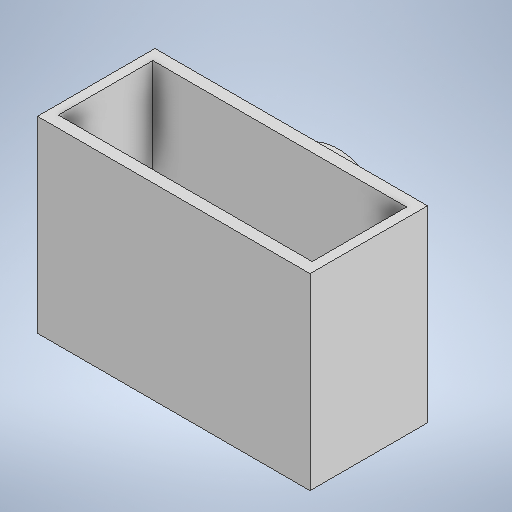
# Autodesk Inventor part: Attache servomoteur_bogie
Saved by Autodesk Inventor 2026.2 (Build 302298010, 298A)
## iProperties
Created: 2026-03-22
Part Number: Attache servomoteur_bogie
Material: Générique
Document SubType Name: Modeling
Designer: Genon
Density: 1 g/cm^3
Appearance: Par défaut
Author: Genon
Autodesk Inventor part; units mm, degrees
ref_plane "YZ Plane" through (0, 0, 0) normal (1, 0, 0) x (0, 1, 0)
ref_plane "XZ Plane" through (0, 0, 0) normal (0, 1, 0) x (-1, 0, 0)
ref_plane "XY Plane" through (0, 0, 0) normal (0, 0, 1) x (1, 0, 0)
sketch "Esquisse1" plane through (0, 0, 0) normal (0, 1, 0) x (-1, 0, 0)
  line L0 (0, 0) -> (0, 2.45)
  line L1 (0, 0) -> (2.45, 0) construction
  line L2 (0, 2.45) -> (27, 2.45)
  line L3 (27, 2.45) -> (27, 22.55)
  line L4 (27, 22.55) -> (-27, 22.55)
  line L5 (-27, 22.55) -> (-27, 2.45)
  line L6 (-27, 2.45) -> (0, 2.45)
  line L7 (0, 0) -> (29, 0)
  line L8 (29, 0) -> (29, 25)
  line L9 (29, 25) -> (-29, 25)
  line L10 (-29, 25) -> (-29, 0)
  line L11 (-29, 0) -> (0, 0)
  dimension "d0" = 2.45
  dimension "d1" = 90
  dimension "d2" = 27
  dimension "d3" = 20.1
  dimension "d4" = 54
  dimension "d5" = 29
  dimension "d6" = 25
  dimension "d7" = 58
  constraints: 24 end point, 6 perpendicular, 4 horizontal, 2 parallel, 1 point on line, 1 vertical
  measures "d0" distance of L0.start L0.end
  measures "d1" angle of L1 L0
  measures "d2" distance of L0.end L2.end
  measures "d3" distance of L2.end L3.end
  measures "d4" distance of L3.end L4.end
  measures "d5" distance of L0.start L7.end
  measures "d6" distance of L7.end L8.end
  measures "d7" distance of L8.end L9.end
extrude "Extrusion1" add sketch "Esquisse1" along normal blind 40
sketch "Esquisse2" plane through (29, 0, 0) normal (0, 0, -1) x (-1, 0, 0)
  line L0 (29, 0) -> (29, 40)
  line L1 (58, 40) -> (0, 40) projected
  line L2 (0, 0) -> (0, 40) projected
  line L3 (0, 20) -> (58, 20)
  line L4 (58, 0) -> (58, 40) projected
  circle A0 centre (29, 20) radius 10
  circle A1 centre (29, 20) radius 11
  dimension "d10" = 20
  dimension "d11" = 22
  constraints: 4 end point, 4 midpoint, 2 centre point, 1 coincident
  measures "d10" diameter of A0
  measures "d11" diameter of A1
extrude "Extrusion2" add sketch "Esquisse2" along normal blind 10 contours A1 L3 A0 L0 | L0 A0 L3 A1 | A1 L0 A0 L3 | L3 A0 L0 A1
sketch "Esquisse3" plane through (0, 0, 0) normal (0, 1, 0) x (-1, 0, 0)
  line L0 (-11, -10) -> (11, -10) projected
  line L1 (0, -10) -> (0, -5)
  point P0 (0, 0)
  dimension "d14" = 5
  constraints: 2 end point, 1 coincident, 1 midpoint, 1 vertical
  measures "d14" distance of L1.start L1.end
hole "Perçage1" at (0, 0, -5) direction (0, 1, 0) diameter 4 end through all
sketch "Esquisse4" plane through (0, 0, 0) normal (0, -1, 0) x (1, 0, 0)
  line L0 (27, 2.45) -> (27, 22.55) projected
  line L1 (27, 22.55) -> (-27, 22.55) projected
  line L2 (-27, 2.45) -> (27, 2.45) projected
  line L3 (-27, 22.55) -> (-27, 2.45) projected
  line L4 (27, 22.55) -> (21, 22.55)
  line L5 (27, 22.55) -> (33, 22.55) construction
  line L6 (21, 22.55) -> (21, 2.45)
  line L7 (-27, 22.55) -> (-21, 22.55)
  line L8 (-21, 22.55) -> (-21, 2.45)
  point P0 (0, 0)
  dimension "d22" = 6
  dimension "d23" = 180
  dimension "d24" = 6
  constraints: 10 end point, 3 point on line, 2 horizontal, 2 perpendicular, 1 collinear
  measures "d22" distance of L0.end L4.end
  measures "d23" angle of L4 L5
  measures "d24" distance of L1.end L7.end
extrude "Extrusion3" add sketch "Esquisse4" against normal blind 16.4 contours L2 L6 L1 L0 | L2 L3 L1 L8
sketch "Esquisse5" plane through (0, 16.4, 0) normal (0, 1, 0) x (1, 0, 0)
  line L0 (-21, -22.55) -> (-21, -2.45) projected
  line L1 (-21, -22.55) -> (-21, -12.5)
  line L2 (-21, -12.5) -> (-21, -11.5)
  line L3 (-27, -22.55) -> (-27, -2.45) projected
  line L4 (-21, -11.5) -> (-27, -11.5)
  line L5 (-21, -12.5) -> (-21, -13.5)
  line L6 (-21, -13.5) -> (-27, -13.5)
  line L7 (0, -14.9752) -> (0, -10.0185)
  line L8 (21, -22.55) -> (21, -2.45)
  line L9 (27, -22.55) -> (27, -2.45)
  line L10 (21, -11.5) -> (27, -11.5)
  line L11 (21, -13.5) -> (27, -13.5)
  point P0 (0, 0)
  dimension "d27" = 10.05
  dimension "d28" = 1
  dimension "d29" = 1
  constraints: 20 end point, 8 symmetric about line, 7 point on line, 2 perpendicular, 1 midpoint, 1 vertical
  measures "d27" distance of L0.start L1.end
  measures "d28" distance of L1.end L2.end
  measures "d29" distance of L1.end L5.end
extrude "Extrusion4" cut sketch "Esquisse5" against normal blind 2
sketch "Esquisse6" plane through (0, 16.4, 0) normal (0, 1, 0) x (1, 0, 0)
  line L0 (-27, -22.55) -> (-27, -2.45) projected
  line L1 (-21, -22.55) -> (-21, -13.5) projected
  line L2 (-21, -11.5) -> (-21, -2.45) projected
  line L3 (-27, -12.5) -> (-27, -17.5)
  line L4 (-27, -17.5) -> (-24.775, -17.5)
  line L5 (-24.775, -17.5) -> (-24.775, -7.5)
  line L6 (0, -16.5029) -> (0, -8.8773)
  point P0 (0, 0)
  point P1 (24.775, -17.5)
  point P2 (24.775, -7.5)
  dimension "d32" = 5
  dimension "d33" = 2.225
  dimension "d34" = 10
  constraints: 8 end point, 2 coincident, 2 perpendicular, 2 symmetric about line, 1 midpoint, 1 point on line, 1 vertical
  measures "d32" distance of L3.start L3.end
  measures "d33" distance of L3.end L4.end
  measures "d34" distance of L4.end L5.end
hole "Perçage2" at (-24.775, 16.4, 17.5) at (-24.775, 16.4, 7.5) at (24.775, 16.4, 17.5) at (24.775, 16.4, 7.5) direction (0, -1, 0) diameter 3.242 depth 11.8 tip angle 118 thread size "M4x0.7" class "6H" standard "ISO Metric profile"
